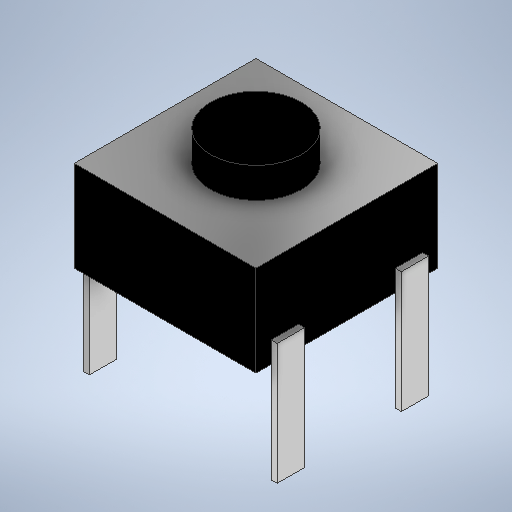
# Autodesk Inventor part: button
Saved by Autodesk Inventor 2025.2 (Build 292293000, 293)
## iProperties
Created: 2025-04-04
Part Number: button
Material: Generic
Document SubType Name: Modeling
Designer: joaki
Density: 1 g/cm^3
Appearance: Default
Author: joaki
Autodesk Inventor part; units mm, degrees
ref_plane "YZ Plane" through (0, 0, 0) normal (1, 0, 0) x (0, 1, 0)
ref_plane "XZ Plane" through (0, 0, 0) normal (0, 1, 0) x (-1, 0, 0)
ref_plane "XY Plane" through (0, 0, 0) normal (0, 0, 1) x (1, 0, 0)
sketch "Sketch1" plane through (0, 0, 0) normal (0, 1, 0) x (-1, 0, 0)
  line L0 (3.3568, 1.5081) -> (-2.6432, 1.5081)
  line L1 (-2.6432, 1.5081) -> (-2.6432, -4.4919)
  line L2 (-2.6432, -4.4919) -> (3.3568, -4.4919)
  line L3 (3.3568, -4.4919) -> (3.3568, 1.5081)
  point P0 (0, 0)
  dimension "d0" = 6
  dimension "d1" = 6
  constraints: 8 end point, 2 parallel, 1 horizontal, 1 perpendicular
  measures "d0" distance of L1.end L2.end
  measures "d1" distance of L2.end L0.start
extrude "Extrusion1" add sketch "Sketch1" along normal blind 3
sketch "Sketch2" plane through (0, 3, 0) normal (0, 1, 0) x (1, 0, 0)
  circle A0 centre (-0.3568, 1.4919) radius 1.5
  line L0 (2.6432, 4.4919) -> (-3.3568, 4.4919) projected
  line L1 (-3.3568, 4.4919) -> (-3.3568, -1.5081) projected
  point P0 (0, 0)
  dimension "d4" = 3
  dimension "d5" = 3
  dimension "d6" = 3
  constraints: 1 centre point
  measures "d4" diameter of A0
  measures "d5" distance from line of L0 A0.centre
  measures "d6" distance from line of L1 A0.centre
extrude "Extrusion2" add sketch "Sketch2" along normal blind 1
sketch "Sketch4" plane through (2.6432, 0, 1.5081) normal (1, 0, 0) x (0, 0, -1)
  line L0 (0, 0) -> (6, 0) projected
  line L1 (0.5, 0) -> (1.4, 0)
  line L2 (1.4, 0) -> (1.4, 0.7)
  line L3 (1.4, 0.7) -> (0.5, 0.7)
  line L4 (0.5, 0.7) -> (0.5, 0)
  line L5 (0.5, 0) -> (1.4, 0)
  line L6 (1.4, 0) -> (1.4, -3.3)
  line L7 (1.4, -3.3) -> (0.5, -3.3)
  line L8 (0.5, -3.3) -> (0.5, 0)
  line L9 (0, 0) -> (0, 3) projected
  line L10 (3, 0) -> (3, 3)
  line L11 (0, 3) -> (6, 3) projected
  line L12 (5.5, 0) -> (4.6, 0)
  line L13 (4.6, 0) -> (4.6, 0.7)
  line L14 (4.6, 0.7) -> (5.5, 0.7)
  line L15 (5.5, 0.7) -> (5.5, 0)
  line L16 (5.5, 0) -> (4.6, 0)
  line L17 (4.6, 0) -> (4.6, -3.3)
  line L18 (4.6, -3.3) -> (5.5, -3.3)
  line L19 (5.5, -3.3) -> (5.5, 0)
  point P0 (1.5081, 0)
  point P1 (1.4, 0.35)
  point P2 (4.4919, 0)
  point P3 (4.6, 0.35)
  dimension "d9" = 0.9
  dimension "d10" = 0.7
  dimension "d11" = 3.3
  dimension "d12" = 0.5
  dimension "d13" = 0
  constraints: 34 end point, 9 symmetric about line, 4 parallel, 3 midpoint, 2 horizontal, 2 perpendicular, 1 point on line
  measures "d9" distance between parallel lines of L2 L4
  measures "d10" distance between parallel lines of L0 L3
  measures "d11" distance between parallel lines of L0 L7
  measures "d12" distance between parallel lines of L9 L4
  measures "d13" distance from line of point (1.4, 0.35) L6
extrude "Extrusion3" add sketch "Sketch4" along normal blind 0.2 contours L13 L14 L15 L0 | L0 L19 L18 L17 | L4 L3 L2 L0 | L0 L6 L7 L8
sketch "Sketch5" plane through (-3.3568, 0, -4.4919) normal (-1, 0, 0) x (0, 0, 1)
  line L0 (0.5, -3.3) -> (0.5, 0.7) projected
  line L1 (1.4, 0.7) -> (1.4, -3.3) projected
  line L2 (0.5, 0.7) -> (1.4, 0.7)
  line L3 (1.4, 0.7) -> (1.4, -3.3)
  line L4 (1.4, -3.3) -> (0.5, -3.3)
  line L5 (0.5, -3.3) -> (0.5, 0.7)
  line L6 (5.5, 0.7) -> (5.5, -3.3) projected
  line L7 (4.6168, 0.7) -> (5.5, 0.7)
  line L8 (5.5, 0.7) -> (5.5, -3.3)
  line L9 (5.5, -3.3) -> (4.6168, -3.3)
  line L10 (4.6168, -3.3) -> (4.6168, 0.7)
  point P0 (4.4919, 0)
  constraints: 16 end point, 4 parallel, 2 horizontal, 2 perpendicular, 1 point on line
extrude "Extrusion4" add sketch "Sketch5" along normal blind 0.2
body "Solid1"
